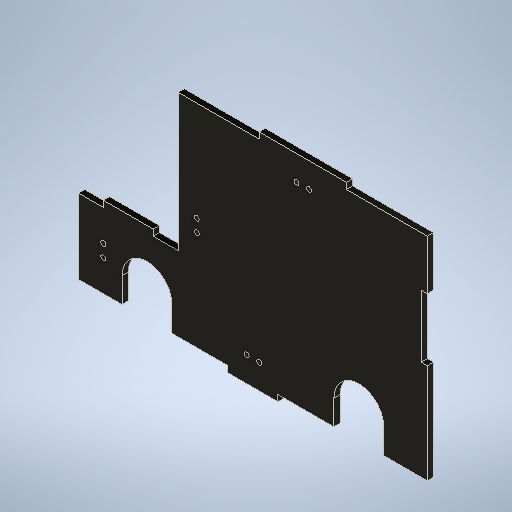
# Autodesk Inventor part: side
Saved by Autodesk Inventor 2025.3 (Build 293356030, 356C)
## iProperties
Created: 2026-06-26
Part Number: side
Material: Generic
Document SubType Name: Modeling
Designer: user
Density: 1 g/cm^3
Appearance: Gunmetal
Author: user
Autodesk Inventor part; units mm, degrees
ref_plane "YZ Plane" through (0, 0, 0) normal (1, 0, 0) x (0, 1, 0)
ref_plane "XZ Plane" through (0, 0, 0) normal (0, 1, 0) x (-1, 0, 0)
ref_plane "XY Plane" through (0, 0, 0) normal (0, 0, 1) x (1, 0, 0)
sketch "Sketch1" plane through (0, 0, 0) normal (0, 0, 1) x (1, 0, 0)
  line L0 (0, 0) -> (0, 60)
  line L1 (0, 60) -> (80, 60)
  line L2 (80, 60) -> (80, 170)
  line L3 (80, 170) -> (280, 170)
  line L4 (280, 170) -> (280, 0)
  line L5 (0, 0) -> (35, 0)
  line L6 (35, 0) -> (35, 20)
  arc A0 (75, 20) -> (35, 20) centre (55, 20) ccw
  line L7 (75, 20) -> (75, 0)
  line L8 (140, 0) -> (140, 170) construction
  line L9 (75, 0) -> (140, 0)
  line L10 (280, 0) -> (245, 0)
  line L11 (245, 0) -> (245, 20)
  arc A1 (245, 20) -> (205, 20) centre (225, 20) ccw
  line L12 (205, 20) -> (205, 0)
  line L13 (205, 0) -> (140, 0)
  line L14 (145, 170) -> (215, 170)
  line L15 (215, 170) -> (215, 175)
  line L16 (215, 175) -> (145, 175)
  line L17 (145, 175) -> (145, 170)
  line L18 (280, 80) -> (275, 80)
  line L19 (275, 80) -> (275, 130)
  line L20 (275, 130) -> (280, 130)
  line L21 (280, 130) -> (280, 80)
  line L22 (10, 20) -> (15, 20)
  line L23 (15, 20) -> (15, 60)
  line L24 (15, 60) -> (10, 60)
  line L25 (10, 60) -> (10, 20)
  line L26 (20, 60) -> (60, 60)
  line L27 (60, 60) -> (60, 65)
  line L28 (60, 65) -> (20, 65)
  line L29 (20, 65) -> (20, 60)
  line L30 (160, 0) -> (160, -5)
  line L31 (160, -5) -> (120, -5)
  line L32 (120, -5) -> (120, 0)
  dimension "d0" = 60
  dimension "d2" = 110
  dimension "d5" = 20
  dimension "d6" = 40
  dimension "d7" = 70
  dimension "d8" = 5
  dimension "d9" = 5
  dimension "d10" = 50
  dimension "d13" = 5
  dimension "d14" = 40
  dimension "d17" = 40
  dimension "d18" = 5
  dimension "d19" = 40
  dimension "d20" = 5
  dimension "d21" = 20
  dimension "d22" = 0
  dimension "d23" = 170
  dimension "d27" = 35
  dimension "d28" = 80
  constraints: 66 end point, 12 perpendicular, 8 parallel, 6 horizontal, 5 point on line, 5 symmetric about line, 4 point on circle, 2 centre point, 2 equal length, 2 tangent, 2 vertical, 1 other
  measures "d0" distance of L0.start L0.end
  measures "d2" distance of L1.end L2.end
  measures "d5" distance of L5.end L6.end
  measures "d6" distance of L6.end L7.start
  measures "d7" distance of L16.end L15.end
  measures "d8" distance of L15.end L14.end
  measures "d9" distance of L19.end L20.end
  measures "d10" distance of L18.end L19.end
  measures "d13" distance of L24.end L23.end
  measures "d14" distance of L23.end L22.end
  measures "d17" distance of L28.end L27.end
  measures "d18" distance of L27.end L26.end
  measures "d19" distance of L30.end L31.end
  measures "d20" distance of L30.start L30.end
  measures "d21" distance between parallel lines of L32 L8
  measures "d22" distance between parallel lines of L4 L21
  measures "d23" distance of A1.centre A0.centre
  measures "d27" distance of L0.start L5.end
  measures "d28" distance of L0.end L1.end
extrude "Extrusion1" add sketch "Sketch1" along normal blind 5 contours L0 L1 L25 L22 L23 L2 L3 L4 L20 L19 L18 L10 L11 A1 L12 L13 L9 L7 A0 L6 L5 | L1 L23 L22 L25 | L29 L28 L27 L1 | L9 L13 L30 L31 L32 | L17 L16 L15 L3
sketch "Sketch2" plane through (0, 0, 5) normal (0, 0, 1) x (1, 0, 0)
  line L0 (215, 175) -> (145, 175) projected
  line L1 (145, 175) -> (145, 170) projected
  line L2 (120, -5) -> (160, -5) projected
  line L3 (160, -5) -> (160, 0) projected
  line L4 (0, 60) -> (0, 0) projected
  line L5 (20, 60) -> (0, 60) projected
  point P0 (175, 155)
  point P1 (185, 155)
  point P2 (135, 15)
  point P3 (145, 15)
  point P4 (20, 35)
  point P5 (20, 25)
  dimension "d43" = 10
  dimension "d44" = 20
  dimension "d45" = 20
  dimension "d46" = 30
  dimension "d47" = 20
  dimension "d48" = 20
  dimension "d49" = 10
  dimension "d50" = 15
  dimension "d51" = 10
  dimension "d52" = 20
  dimension "d53" = 20
  dimension "d54" = 25
  measures "d43" distance of point (185, 155) point (175, 155)
  measures "d44" distance from line of point (185, 155) L0
  measures "d45" distance from line of L0 point (175, 155)
  measures "d46" distance from line of L1 point (175, 155)
  measures "d47" distance from line of L2 point (135, 15)
  measures "d48" distance from line of L2 point (145, 15)
  measures "d49" distance of point (145, 15) point (135, 15)
  measures "d50" distance from line of L3 point (145, 15)
  measures "d51" distance of point (20, 25) point (20, 35)
  measures "d52" distance from line of L4 point (20, 25)
  measures "d53" distance from line of L4 point (20, 35)
  measures "d54" distance from line of point (20, 35) L5
hole "Hole1" at (175, 155, 5) at (185, 155, 5) at (135, 15, 5) at (145, 15, 5) at (20, 35, 5) at (20, 25, 5) direction (0, 0, -1) diameter 4 end through all
sketch "Sketch4" plane through (0, 0, 5) normal (0, 0, 1) x (1, 0, 0)
  line L0 (80, 170) -> (80, 60) projected
  line L1 (80, 60) -> (60, 60) projected
  point P0 (0, 0)
  point P1 (95, 80)
  point P2 (95, 90)
  dimension "d63" = 15
  dimension "d64" = 15
  dimension "d65" = 10
  dimension "d66" = 20
  measures "d63" distance from line of point (95, 80) L0
  measures "d64" distance from line of L0 point (95, 90)
  measures "d65" distance of point (95, 80) point (95, 90)
  measures "d66" distance from line of L1 point (95, 80)
hole "Hole3" at (95, 80, 5) at (95, 90, 5) direction (0, 0, -1) diameter 4 end through all
body "Solid1"
